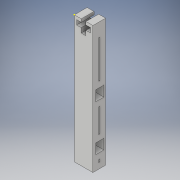
# Autodesk Inventor part: ripnewvertical2
Saved by Autodesk Inventor 2017 (Build 210142000, 142)
## iProperties
Created: 2017-11-22
Part Number: ripnewvertical2
Material: Generic
Document SubType Name: Modeling
Designer: build
Density: 1 g/cm^3
Appearance: Default
Author: build
Autodesk Inventor part; units mm, degrees
ref_plane "YZ Plane" through (0, 0, 0) normal (1, 0, 0) x (0, 1, 0)
ref_plane "XZ Plane" through (0, 0, 0) normal (0, 1, 0) x (-1, 0, 0)
ref_plane "XY Plane" through (0, 0, 0) normal (0, 0, 1) x (1, 0, 0)
sketch "Sketch1" plane through (0, 0, 0) normal (0, 0, 1) x (1, 0, 0)
  line L0 (0, 0) -> (20.32, 0)
  line L1 (20.32, 0) -> (20.32, -139.7)
  line L2 (20.32, -139.7) -> (0, -139.7)
  line L3 (0, -139.7) -> (0, 0)
  line L4 (0, 0) -> (7.62, 0)
  line L5 (20.32, 0) -> (12.7, 0)
  line L6 (7.62, 0) -> (7.62, -3.302)
  line L7 (12.7, 0) -> (12.7, -3.302)
  line L8 (12.7, -3.302) -> (17.78, -3.302)
  line L9 (17.78, -3.302) -> (17.78, -8.382)
  line L10 (17.78, -8.382) -> (12.7, -8.382)
  line L11 (12.7, -8.382) -> (12.7, -13.462)
  line L12 (12.7, -13.462) -> (7.62, -13.462)
  line L13 (7.62, -13.462) -> (7.62, -8.382)
  line L14 (7.62, -8.382) -> (2.54, -8.382)
  line L15 (2.54, -8.382) -> (2.54, -3.302)
  line L16 (2.54, -3.302) -> (7.62, -3.302)
  line L17 (7.62, -3.302) -> (7.62, 0)
  dimension "d0" = 20.32
  dimension "d1" = 139.7
  dimension "d2" = 7.62
  dimension "d3" = 7.62
  dimension "d4" = 3.302
  dimension "d5" = 5.08
  dimension "d6" = 5.08
  dimension "d7" = 5.08
  dimension "d8" = 5.08
  dimension "d9" = 5.08
  dimension "d10" = 5.08
  dimension "d11" = 5.08
  dimension "d12" = 5.08
  dimension "d13" = 5.08
  constraints: 36 end point, 7 point on line, 4 perpendicular, 3 parallel, 2 vertical, 1 collinear, 1 horizontal
  measures "d0" distance of L0.start L0.end
  measures "d1" distance of L0.end L1.end
  measures "d2" distance of L0.start L4.end
  measures "d3" distance of L0.end L5.end
  measures "d4" distance of L4.end L6.end
  measures "d5" distance of L7.end L8.end
  measures "d6" distance of L8.end L9.end
  measures "d7" distance of L9.end L10.end
  measures "d8" distance of L10.end L11.end
  measures "d9" distance of L11.end L12.end
  measures "d10" distance of L12.end L13.end
  measures "d11" distance of L13.end L14.end
  measures "d12" distance of L14.end L15.end
  measures "d13" distance of L15.end L6.end
extrude "Extrusion1" add sketch "Sketch1" along normal blind 13.97 contours L0 L6 L16 L15 L14 L13 L12 L11 L10 L9 L8 L7 L1 L2 L3
sketch "Sketch2" plane through (20.32, -139.7, 0) normal (1, 0, 0) x (0, 0, -1)
  line L0 (-10.7501, 15.4155) -> (-10.7501, 26.5915)
  line L1 (-10.7501, 26.5915) -> (-1.8601, 26.5915)
  line L2 (-1.8601, 26.5915) -> (-1.8601, 15.4155)
  line L3 (-1.8601, 15.4155) -> (-10.7501, 15.4155)
  line L4 (-10.7501, 65.6672) -> (-10.7501, 77.0972)
  line L5 (-10.7501, 77.0972) -> (-1.8601, 77.0972)
  line L6 (-1.8601, 77.0972) -> (-1.8601, 65.6672)
  line L7 (-1.8601, 65.6672) -> (-10.7501, 65.6672)
  point P0 (0, 139.7)
  dimension "d16" = 11.176
  dimension "d17" = 8.89
  dimension "d18" = 11.43
  dimension "d19" = 8.89
  constraints: 16 end point, 4 parallel, 2 perpendicular, 2 vertical
  measures "d16" distance of L0.start L0.end
  measures "d17" distance of L0.end L1.end
  measures "d18" distance of L4.start L4.end
  measures "d19" distance of L4.end L5.end
extrude "Extrusion2" cut sketch "Sketch2" against normal blind 533.4
shell "Shell1" thickness 6.35 removed faces 1 at (20.32, -20.8676, 8.24)
sketch "Sketch3" plane through (0, 0, 13.97) normal (0, 0, 1) x (1, 0, 0)
  point P0 (0, 0)
body "Solid1"
